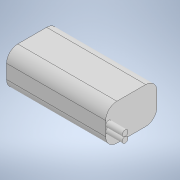
# Autodesk Inventor part: Battery
Saved by Autodesk Inventor 2022 (Build 260153000, 153)
## iProperties
Created: 2022-08-09
Part Number: Battery
Material: Generic
Document SubType Name: Modeling
Designer: Nick
Density: 1 g/cm^3
Appearance: Default
Author: Nick
Autodesk Inventor part; units mm, degrees
ref_plane "YZ Plane" through (0, 0, 0) normal (1, 0, 0) x (0, 1, 0)
ref_plane "XZ Plane" through (0, 0, 0) normal (0, 1, 0) x (-1, 0, 0)
ref_plane "XY Plane" through (0, 0, 0) normal (0, 0, 1) x (1, 0, 0)
sketch "Sketch1" plane through (0, 0, 0) normal (1, 0, 0) x (0, 1, 0)
  line L0 (0, 0) -> (22, 0)
  line L1 (22, 0) -> (22, -31)
  line L2 (22, -31) -> (0, -31)
  line L3 (0, -31) -> (0, 0)
  dimension "d0" = 22
  dimension "d1" = 31
  constraints: 8 end point, 2 parallel, 1 horizontal, 1 perpendicular
  measures "d0" distance of L1.end L2.end
  measures "d1" distance of L0.end L1.end
extrude "Extrusion1" add sketch "Sketch1" along normal blind 60
sketch "Sketch2" plane through (60, 0, 0) normal (1, 0, 0) x (0, 0, -1)
  circle A0 centre (1.75, 9.25) radius 1.75
  circle A1 centre (1.75, 12.75) radius 1.75
  line L0 (1.75, 9.25) -> (1.75, 12.75) construction
  line L1 (0, 22) -> (0, 0) projected
  point P0 (1.75, 11)
  point P1 (0, 11)
  point P2 (1.75, 11)
  dimension "d4" = 3.5
  constraints: 2 centre point, 2 end point, 2 midpoint, 2 tangent, 1 equal radius, 1 horizontal alignment, 1 vertical, 1 vertical alignment
  measures "d4" diameter of A1
extrude "Extrusion2" add sketch "Sketch2" along normal blind 10 contours A0 | A1
fillet "Fillet1" radius 6.7625 4 edges at (30, 0, 0) (30, 22, 0) (30, 0, -31) (30, 22, -31)
body "Solid1"
